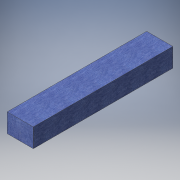
# Autodesk Inventor part: Bumper
Saved by Autodesk Inventor 2016 (Build 200138000, 138)
## iProperties
Created: 2016-01-26
Part Number: Bumper
Material: Generic
Document SubType Name: Modeling
Designer: ares-b02
Density: 1 g/cm^3
Appearance: Denim - Blue
Author: ares-b02
Autodesk Inventor part; units mm, degrees
ref_plane "YZ Plane" through (0, 0, 0) normal (1, 0, 0) x (0, 1, 0)
ref_plane "XZ Plane" through (0, 0, 0) normal (0, 1, 0) x (-1, 0, 0)
ref_plane "XY Plane" through (0, 0, 0) normal (0, 0, 1) x (1, 0, 0)
sketch "Sketch1" plane through (0, 0, 0) normal (0, 0, 1) x (1, 0, 0)
  line L0 (-8.0757, 4.9663) -> (106.2243, 4.9663)
  line L1 (106.2243, 4.9663) -> (106.2243, -77.5837)
  line L2 (106.2243, -77.5837) -> (-8.0757, -77.5837)
  line L3 (-8.0757, -77.5837) -> (-8.0757, 4.9663)
  point P0 (0, 0)
  dimension "d0" = 114.3
  dimension "d1" = 82.55
  constraints: 8 end point, 2 parallel, 1 horizontal, 1 perpendicular
  measures "d0" distance of L0.start L0.end
  measures "d1" distance of L2.end L0.start
extrude "Extrusion1" add sketch "Sketch1" along normal blind 609.6
body "Solid1"
